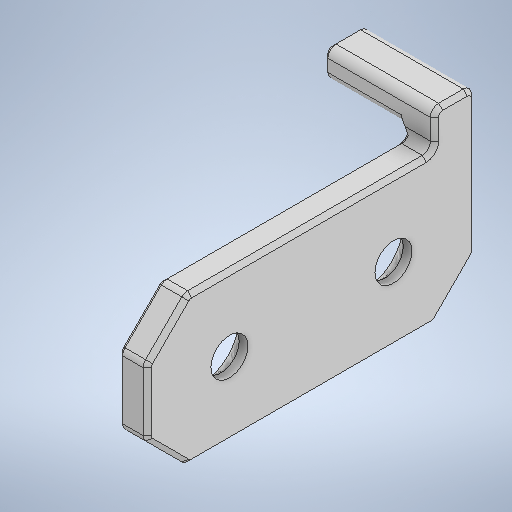
# Autodesk Inventor part: Kopf
Saved by Autodesk Inventor 2025.1 (Build 291241000, 241)
## iProperties
Created: 2024-11-26
Part Number: Kopf
Material: Generisch
Document SubType Name: Modeling
Designer: Kai Altwicker
Density: 1 g/cm^3
Appearance: Vorgabe
Author: Kai Altwicker
Autodesk Inventor part; units mm, degrees
ref_plane "YZ Plane" through (0, 0, 0) normal (1, 0, 0) x (0, 1, 0)
ref_plane "XZ Plane" through (0, 0, 0) normal (0, 1, 0) x (-1, 0, 0)
ref_plane "XY Plane" through (0, 0, 0) normal (0, 0, 1) x (1, 0, 0)
sketch "Skizze1" plane through (0, 0, 0) normal (1, 0, 0) x (0, 1, 0)
  line L0 (9, 20) -> (-9, 20)
  line L1 (-9, 20) -> (-9, -20)
  line L2 (-9, -20) -> (9, -20)
  line L3 (9, -20) -> (9, 20)
  point P0 (0, 0)
  point P1 (-9, 0)
  point P2 (0, -20)
  dimension "d0" = 18
  dimension "d1" = 40
  constraints: 8 end point, 2 midpoint, 2 parallel, 1 horizontal, 1 horizontal alignment, 1 perpendicular, 1 vertical alignment
  measures "d0" distance of L1.end L2.end
  measures "d1" distance of L0.end L1.end
extrude "Extrusion1" add sketch "Skizze1" along normal blind 3.5
sketch "Skizze2" plane through (0, -9, -20) normal (0, 0, -1) x (-1, 0, 0)
  line L0 (0, 18) -> (-3.5, 18) projected
  line L1 (0, 18) -> (0, 19)
  line L2 (0, 19) -> (10, 19)
  line L3 (10, 19) -> (10, 22.5)
  line L4 (10, 22.5) -> (-3.5, 22.5)
  line L5 (-3.5, 22.5) -> (-3.5, 18)
  line L6 (0, 0) -> (0, 18) projected
  line L7 (-3.5, 0) -> (-3.5, 18) projected
  point P0 (0, 9)
  point P1 (0, 9)
  dimension "d4" = 10
  dimension "d5" = 3.5
  dimension "d6" = 10
  constraints: 10 end point, 3 perpendicular, 1 collinear, 1 midpoint
  measures "d4" distance from line of L2 point (0, 9)
  measures "d5" distance between parallel lines of L4 L2
  measures "d6" distance of L1.end L2.end
extrude "Extrusion2" add sketch "Skizze2" against normal blind 5
chamfer "Fasen1" distance 5 angle 45 3 edges at (1.75, 9, 20) (1.75, -9, 20) (1.75, -9, -20)
fillet "Rundung1" radius 1 11 edges at (-3.25, 13.5, -15) (-5, 10, -15) (1.75, 9, -15) (-3.25, 13.5, -20) (1.75, -4, -20) (1.75, -9, -15) (1.75, -9, 15) (1.75, -4, 20) (1.75, 4, 20) (1.75, 9, 15) (-5, 10, -20)
sketch "Skizze3" plane through (0, 0, 0) normal (-1, 0, 0) x (0, 0, 1)
  line L0 (20, 3.5858) -> (20, -3.5858) projected
  point P0 (0, 0)
  point P1 (10, 0)
  point P2 (-10, 0)
  point P3 (20, 0)
  dimension "d13" = 10
  dimension "d14" = 20
  constraints: 2 horizontal alignment, 1 midpoint
  measures "d13" distance from line of L0 point (10, 0)
  measures "d14" distance of point (10, 0) point (-10, 0)
hole "Bohrung1" at (0, 0, -10) at (0, 0, 10) direction (1, 0, 0) diameter 4.5 end through all countersink diameter 9.4 countersink angle 90 clearance for "Flachkopfsenkschraube DIN EN ISO 2009" size "M4" standard "DIN"
chamfer "Fasen2" distance 0.5 angle 45 3 edges at (0, 10, -17.5) (0, 10.2929, -15.2929) (0, 10.2929, -19.7071)
chamfer "Fasen3" distance 0.5 angle 45 40 edges at (0, 9, 0.2929) (0, 8.9239, 14.9685) (0, 6.5, 17.5) (0, 3.9685, 19.9239) (0, 0, 20) (0, -3.9685, 19.9239) (0, -6.5, 17.5) (0, -8.9239, 14.9685) (0, -9, 0) (0, -8.9239, -14.9685) (0, -6.5, -17.5) (0, -3.9685, -19.9239) (0, 3.148, -20) (0, 9.2542, -14.6663) (-10, 10, -17.5) (-10, 10.2929, -15.2929) (-10, 11.75, -15) (-10, 13.2071, -15.2929) (-10, 13.5, -17.5) (-10, 13.2071, -19.7071) (-10, 11.75, -20) (-10, 10.2929, -19.7071) (3.5, 9, 0.2929) (3.5, 8.9239, 14.9685) (3.5, 6.5, 17.5) (3.5, 3.9685, 19.9239) (3.5, 0, 20) (3.5, -3.9685, 19.9239) (3.5, -6.5, 17.5) (3.5, -8.9239, 14.9685) (3.5, -9, 0) (3.5, -8.9239, -14.9685) (3.5, -6.5, -17.5) (3.5, -3.9685, -19.9239) (3.5, 4.4571, -20) (3.5, 13.2071, -19.7071) (3.5, 13.5, -17.5) (3.5, 13.2071, -15.2929) (3.5, 11.25, -15) (3.5, 9.2929, -14.7071)
equation "\"d_tol\" = 0.3"
equation "\"d_wand\" = 1.5"
equation "\"b_rasp_pi\" = 56"
equation "\"w_kamera_hori\" = 66deg"
equation "\"l_rasp_pi\" = 85"
equation "\"w_kamera_vert\" = 41deg"
equation "\"r_rasp_pi\" = 3"
equation "\"D_oct\" = 3621.32034"
equation "\"D_hexadeca\" = 7541.00924"
equation "\"d_traeger\" = 625"
